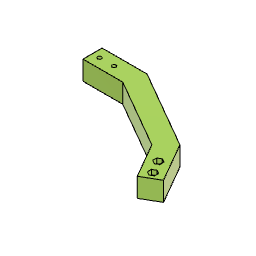
circular_frame (Autodesk Fusion 360 design; units mm, degrees)
Autodesk Fusion 360 part; units mm, degrees
sketch "Sketch1" plane through (0, 0, 0) normal (0, 0, 1) x (1, 0, 0)
  line L0 (151.5544, -62.5) -> (128.1089, -21.8911)
  line L1 (128.1089, -21.8911) -> (46.8911, 25)
  line L2 (46.8911, 25) -> (0, 25)
  line L3 (0, 0) -> (0, 25)
  arc A0 (129.9038, -75) -> (0, 0) centre (0, -150) ccw
  line L4 (151.5544, -62.5) -> (129.9038, -75)
  line L5 (113.4679, -36.5321) -> (41.5321, 5)
  line L6 (41.5321, 5) -> (0, 5)
  line L7 (134.2339, -72.5) -> (113.4679, -36.5321)
  line L8 (77.5, -15.7661) -> (87.5, 1.5544)
  point P0 (0, -150)
  point P1 (0, -150)
  dimension "d1" = 300
  dimension "d4" = 150
  dimension "d5" = 150
  dimension "d14" = 25
  dimension "d15" = 25
  dimension "d16" = 60
  dimension "d17" = 175
  dimension "d30" = 20
  dimension "d31" = 20
  dimension "d32" = 20
  constraint coincident L3.start A0
  constraint vertical L3.start A0.centre
  constraint coincident P0 A0.centre
  constraint horizontal L2
  constraint coincident L3.start A0.end
  constraint coincident L3 A0.end
  constraint collinear L3.start P1 L2.end
  constraint collinear P0 L0.start A0.start
  constraint coincident L3 L6.end
  constraint perpendicular L3 L6
  constraint parallel L1 L5
  constraint midpoint L5 L8.start
  constraint midpoint L1 L8.end
  measures "d1" diameter of A0
  measures "d4" angle of L1 L2
  measures "d5" angle of L0 L1
  measures "d14" distance of L3.start L2.end
  measures "d15" distance of L0.start A0.start
  measures "d16" angle of L3 L4
  measures "d17" distance of P0 L1
  measures "d30" distance of L0 L7
  measures "d31" distance of L2.end L6.end
  measures "d32" distance of L1 L5
extrude "Extrude1" add sketch "Sketch1" along normal blind 20 contours L1 L2 L3 L5 L6 L8
mirror "Mirror2" about plane through (77.5, -15.7661, 0) normal (-0.866025, 0.5, 0) of bodies 1 merged
sketch "Sketch4" plane through (0, 0, 20) normal (0, 0, 1) x (-1, 0, 0)
  line L0 (-128.1089, 21.8911) -> (-46.8911, -25)
  line L1 (-46.8911, -25) -> (0, -25)
  line L2 (-41.5321, -5) -> (-41.5321, -25) construction
  line L3 (-41.5321, -15) -> (0, -15) construction
  circle A0 centre (-7.5, -15) radius 2
  circle A1 centre (-22.5, -15) radius 2
  line L4 (-3.8, -17.1362) -> (-3.8, -12.8638)
  line L5 (-3.8, -12.8638) -> (-7.5, -10.7276)
  line L6 (-7.5, -10.7276) -> (-11.2, -12.8638)
  line L7 (-11.2, -12.8638) -> (-11.2, -17.1362)
  line L8 (-11.2, -17.1362) -> (-7.5, -19.2724)
  line L9 (-7.5, -19.2724) -> (-3.8, -17.1362)
  line L10 (-18.8, -17.1362) -> (-18.8, -12.8638)
  line L11 (-18.8, -12.8638) -> (-22.5, -10.7276)
  line L12 (-22.5, -10.7276) -> (-26.2, -12.8638)
  line L13 (-26.2, -12.8638) -> (-26.2, -17.1362)
  line L14 (-26.2, -17.1362) -> (-22.5, -19.2724)
  line L15 (-22.5, -19.2724) -> (-18.8, -17.1362)
  line L16 (0, -5) -> (-41.5321, -5)
  line L17 (-41.5321, -5) -> (-113.4679, 36.5321)
  line L18 (0, -25) -> (0, -5)
  line L19 (-113.4679, 36.5321) -> (-134.2339, 72.5)
  line L20 (-134.2339, 72.5) -> (-151.5544, 62.5)
  line L21 (-151.5544, 62.5) -> (-128.1089, 21.8911)
  line L22 (-77.5, 15.7661) -> (-87.5, -1.5544) construction
  line L23 (-142.8442, 58.8686) -> (-142.8442, 63.141)
  line L24 (-139.1442, 56.7324) -> (-142.8442, 58.8686)
  line L25 (-135.4442, 58.8686) -> (-139.1442, 56.7324)
  line L26 (-135.4442, 63.141) -> (-135.4442, 58.8686)
  line L27 (-139.1442, 65.2772) -> (-135.4442, 63.141)
  line L28 (-142.8442, 63.141) -> (-139.1442, 65.2772)
  line L29 (-131.6442, 52.2868) -> (-127.9442, 50.1506)
  line L30 (-135.3442, 50.1506) -> (-131.6442, 52.2868)
  line L31 (-135.3442, 45.8782) -> (-135.3442, 50.1506)
  line L32 (-131.6442, 43.742) -> (-135.3442, 45.8782)
  line L33 (-127.9442, 45.8782) -> (-131.6442, 43.742)
  line L34 (-127.9442, 50.1506) -> (-127.9442, 45.8782)
  circle A2 centre (-139.1442, 61.0048) radius 2
  circle A3 centre (-131.6442, 48.0144) radius 2
  point P0 (-7.5, -15)
  point P1 (-22.5, -15)
  dimension "d18" = 4
  dimension "d19" = 7.5
  dimension "d20" = 15
  dimension "d21" = 7.4
  constraint coincident L1 L2.end
  constraint perpendicular L1 L2
  constraint midpoint L2 L3.start
  constraint coincident L3 P0
  constraint coincident L3 P1
  constraint equal A0 A1
  constraint coincident P0 A0.centre
  constraint coincident P1 A1.centre
  constraint vertical L4
  constraint vertical L10
  constraint horizontal L8.end L14.end
  constraint horizontal L3
  constraint coincident L2.start L16
  constraint coincident L3.end L18
  constraint coincident L2.start L16.end
  constraint midpoint L17 L22.start
  constraint midpoint L0 L22.end
  constraint symmetric L4.start L22 L23.end
  constraint symmetric L4.end L22 L27.start
  constraint symmetric L5.end L22 L26.start
  constraint symmetric L6.end L22 L25.start
  constraint symmetric L7.end L22 L24.start
  constraint symmetric L8.end L22 L23.start
  constraint symmetric L10.start L22 L30.start
  constraint symmetric L10.end L22 L29.start
  constraint symmetric L11.end L22 L29.end
  constraint symmetric L12.end L22 L33.start
  constraint symmetric L13.end L22 L32.start
  constraint symmetric L14.end L22 L31.start
  constraint symmetric A0 L22 A2
  constraint symmetric A1 L22 A3
  measures "d18" diameter of A0
  measures "d19" distance of L3.end P0
  measures "d20" distance of P0 P1
  measures "d21" distance of L4 L7
extrude "Extrude4" cut sketch "Sketch4" against normal through all contours A0 | A1 | A2 | A3
extrude "Extrude5" cut sketch "Sketch4" along normal blind 5 from surface at -20 contours L4 L5 L6 L7 L8 L9 | L10 L11 L12 L13 L14 L15
extrude "Extrude6" cut sketch "Sketch4" against normal blind 5 contours L23 L24 L25 L26 L27 L28 | L29 L30 L31 L32 L33 L34
equation "d21 = 7 mm + 2 * gap"
equation "gap = 0.2 mm"
